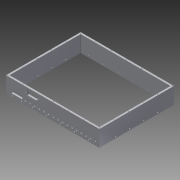
# Autodesk Inventor part: R58010-175-with SNAP V2 features
Saved by Autodesk Inventor 2016 (Build 200138000, 138)
## iProperties
Created: 2014-01-15
Part Number: R58010-175-with SNAP V2 features
Material: Aluminum 6061
Document SubType Name: Modeling
Designer: rtreacy
Density: 1 g/cm^3
Appearance: Aluminum - Flat
Author: rtreacy
Autodesk Inventor part; units mm, degrees
note: some values were not read from the file. Chosen so that the rebuilt part matches the saved one: direction of "Hole23".
ref_plane "YZ Plane" through (0, 0, 0) normal (1, 0, 0) x (0, 1, 0)
ref_plane "XZ Plane" through (0, 0, 0) normal (0, 1, 0) x (-1, 0, 0)
ref_plane "XY Plane" through (0, 0, 0) normal (0, 0, 1) x (1, 0, 0)
sketch "Ext-Sketch" plane through (0, 0, 0) normal (0, 1, 0) x (-1, 0, 0)
  line L0 (-60.3663, -75.973) -> (184.1341, -75.973)
  line L1 (184.1341, -75.973) -> (184.1341, -269.6734)
  line L2 (184.1341, -269.6734) -> (-60.3663, -269.6734)
  line L3 (-60.3663, -269.6734) -> (-60.3663, -75.973)
  line L4 (188.8839, -274.4232) -> (-65.1161, -274.4232)
  line L5 (-65.1161, -274.4232) -> (-65.1161, -71.2232)
  line L6 (-65.1161, -71.2232) -> (188.8839, -71.2232)
  line L7 (188.8839, -71.2232) -> (188.8839, -274.4232)
  point P0 (0, 0)
  dimension "d6" = 244.5004
  dimension "d8" = 193.7004
  dimension "d9" = 203.2
  dimension "d10" = 254
  dimension "d11" = 4.7498
  dimension "d12" = 4.7498
  constraints: 16 end point, 4 parallel, 2 horizontal, 2 perpendicular
  measures "d6" distance of L0.start L0.end
  measures "d8" distance of L0.end L1.end
  measures "d9" distance of L6.end L4.start
  measures "d10" distance of L4.start L4.end
  measures "d11" horizontal distance of L0.start L5.end
  measures "d12" horizontal distance of L6.end L0.end
extrude "Extrusion1" add sketch "Ext-Sketch" along normal blind 44.45
sketch "left-2" plane through (-188.8839, 0, -274.4232) normal (-1, 0, 0) x (0, 0, 1)
  circle A0 centre (19.3548, 11.938) radius 2.1971 projected
  line L0 (203.2, 0) -> (0, 0) projected
  line L1 (203.2, 0) -> (203.2, 44.45) projected
  line L2 (0, 44.45) -> (203.2, 44.45) projected
  line L3 (0, 0) -> (0, 44.45) projected
  point P0 (274.4232, 0)
sketch "left-1" plane through (-188.8839, 0, -274.4232) normal (-1, 0, 0) x (0, 0, 1)
  line L0 (4.7498, 0) -> (4.7498, 44.45) projected
  point P0 (274.4232, 0)
  point P1 (203.2, 0)
  point P2 (203.2, 44.45)
  point P3 (158.75, 4.699)
  dimension "d260" = 44.45
  dimension "d261" = 4.699
  measures "d260" horizontal distance of point (203.2, 44.45) point (158.75, 4.699)
  measures "d261" vertical distance of point (203.2, 0) point (158.75, 4.699)
sketch "bottom-1" plane through (0, 0, 0) normal (0, -1, 0) x (1, 0, 0)
  point P0 (-188.8839, -71.2232)
  point P1 (0, 0)
  point P2 (-186.509, -73.5981)
  point P3 (65.1161, -274.4232)
  point P4 (62.7412, -272.0483)
  dimension "d125" = 2.3749
  dimension "d126" = 2.3749
  dimension "d140" = 2.3749
  dimension "d141" = 2.3749
  measures "d125" horizontal distance of point (-188.884, -71.223) point (-186.509, -73.598)
  measures "d126" horizontal distance of point (-188.884, -71.223) point (-186.509, -73.598)
  measures "d140" horizontal distance of point (65.116, -274.423) point (62.741, -272.048)
  measures "d141" horizontal distance of point (65.116, -274.423) point (62.741, -272.048)
hole "Hole8" at (-186.509, 0, -73.5981) direction (0, 1, 0) diameter 1.7018 depth 5.08 tip angle 118
hole "Hole9" at (62.7412, 0, -272.0483) direction (0, 1, 0) diameter 1.7018 depth 5.08 tip angle 118
sketch "front-1" plane through (-188.8839, 0, -71.2232) normal (0, 0, 1) x (1, 0, 0)
  circle A0 centre (52.07, 10.414) radius 2.159
  line L0 (254, 0) -> (254, 44.45) projected
  line L1 (14.2748, 19.746) -> (14.2748, 9.3472)
  line L2 (14.2748, 9.3472) -> (43.975, 9.3472)
  line L3 (43.975, 9.3472) -> (43.975, 19.746)
  line L4 (43.975, 19.746) -> (14.2748, 19.746)
  line L5 (0, 44.45) -> (254, 44.45) projected
  circle A1 centre (64.77, 10.414) radius 2.159
  circle A2 centre (77.47, 10.414) radius 2.159
  circle A3 centre (90.17, 10.414) radius 2.159
  circle A4 centre (102.87, 10.414) radius 2.159
  circle A5 centre (115.57, 10.414) radius 2.159
  circle A6 centre (128.27, 10.414) radius 2.159
  circle A7 centre (140.97, 10.414) radius 2.159
  circle A8 centre (153.67, 10.414) radius 2.159
  circle A9 centre (166.37, 10.414) radius 2.159
  circle A10 centre (179.07, 10.414) radius 2.159
  circle A11 centre (191.77, 10.414) radius 2.159
  circle A12 centre (204.47, 10.414) radius 2.159
  circle A13 centre (217.17, 10.414) radius 2.159
  circle A14 centre (229.87, 10.414) radius 2.159
  circle A15 centre (242.57, 10.414) radius 2.159
  point P0 (16.51, 4.699)
  point P1 (52.07, 16.51)
  point P2 (0, 0)
  point P3 (52.07, 4.318)
  point P4 (64.77, 16.51)
  point P5 (64.77, 4.318)
  point P6 (77.47, 16.51)
  point P7 (77.47, 4.318)
  point P8 (90.17, 16.51)
  point P9 (90.17, 4.318)
  point P10 (102.87, 16.51)
  point P11 (102.87, 4.318)
  point P12 (115.57, 16.51)
  point P13 (115.57, 4.318)
  point P14 (128.27, 16.51)
  point P15 (128.27, 4.318)
  point P16 (140.97, 16.51)
  point P17 (140.97, 4.318)
  point P18 (153.67, 16.51)
  point P19 (153.67, 4.318)
  point P20 (166.37, 16.51)
  point P21 (166.37, 4.318)
  point P22 (179.07, 16.51)
  point P23 (179.07, 4.318)
  point P24 (191.77, 16.51)
  point P25 (191.77, 4.318)
  point P26 (204.47, 16.51)
  point P27 (204.47, 4.318)
  point P28 (217.17, 16.51)
  point P29 (217.17, 4.318)
  point P30 (229.87, 16.51)
  point P31 (229.87, 4.318)
  point P32 (242.57, 16.51)
  point P33 (242.57, 4.318)
  point P34 (71.12, 4.699)
  dimension "d197" = 6.096
  dimension "d203" = 12.192
  dimension "d222" = 29.7002
  dimension "d223" = 10.3988
  dimension "d224" = 52.07
  dimension "d225" = 10.414
  dimension "d227" = 9.3472
  dimension "d259" = 4.699
  dimension "d273" = 12.7
  dimension "d299" = 14.2748
  dimension "d300" = 52.07
  dimension "d301" = 52.07
  dimension "d302" = 16.51
  dimension "d306" = 6.35
  dimension "d307" = 4.699
  dimension "d434" = 4.318
  constraints: 16 centre point, 8 end point, 3 parallel, 1 horizontal, 1 perpendicular, 60 other
  measures "d197" distance of point (52.07, 16.51) A0.centre
  measures "d203" distance of point (52.07, 16.51) point (52.07, 4.318)
  measures "d222" distance of L3.end L1.start
  measures "d223" distance of L2.end L3.end
  measures "d224" horizontal distance of L5.start A0.centre
  measures "d225" vertical distance of point (0, 0) A0.centre
  measures "d227" vertical distance of L0.start L2.end
  measures "d259" vertical distance of L0.start point (16.51, 4.699)
  measures "d273" distance of point (52.07, 16.51) point (64.77, 16.51)
  measures "d299" horizontal distance of L1.start L5.start
  measures "d300" horizontal distance of point (52.07, 16.51) L5.start
  measures "d301" horizontal distance of point (52.07, 4.318) L5.start
  measures "d302" horizontal distance of point (16.51, 4.699) point (0, 0)
  measures "d306" horizontal distance of point (71.12, 4.699) A1.centre
  measures "d307" vertical distance of point (0, 0) point (71.12, 4.699)
  measures "d434" diameter of A2
hole "Hole10" at (-172.3739, 4.699, -71.2232) direction (0, 0, -1) diameter 2.4384 depth 25.4 tip angle 118 countersink diameter 4.064 countersink angle 82
sketch "right-1" plane through (65.1161, 0, -71.2232) normal (1, 0, 0) x (0, 0, -1)
  point P0 (-71.2232, 0)
  point P1 (158.75, 4.699)
  point P2 (0, 0)
  point P3 (203.2, 44.45)
  dimension "d254" = 44.45
  dimension "d255" = 4.699
  measures "d254" horizontal distance of point (203.2, 44.45) point (158.75, 4.699)
  measures "d255" vertical distance of point (0, 0) point (158.75, 4.699)
hole "Hole11" at (65.1161, 4.699, -229.9732) direction (-1, 0, 0) diameter 2.4384 depth 25.4 tip angle 118 countersink diameter 4.064 countersink angle 82
sketch "back-1" plane through (65.1161, 0, -274.4232) normal (0, 0, -1) x (-1, 0, 0)
  point P0 (65.1161, 0)
  point P1 (228.6, 4.699)
  point P2 (254, 0)
  point P3 (254, 44.45)
  dimension "d256" = 25.4
  dimension "d257" = 4.699
  measures "d256" horizontal distance of point (254, 44.45) point (228.6, 4.699)
  measures "d257" vertical distance of point (254, 0) point (228.6, 4.699)
hole "Hole12" at (-163.4839, 4.699, -274.4232) direction (0, 0, 1) diameter 2.4384 depth 25.4 tip angle 118 countersink diameter 4.064 countersink angle 82
pattern_linear "Rectangular Pattern9" count 6 spacing 39.6748 along (0, 0, -1) of "Hole8"
pattern_linear "Rectangular Pattern10" count 7 spacing 41.529 along (1, 0, 0) of "Hole8"
pattern_linear "Rectangular Pattern11" count 6 spacing 39.6748 along (0, 0, 1) of "Hole9"
pattern_linear "Rectangular Pattern12" count 7 spacing 41.529 along (-1, 0, 0) of "Hole9"
sketch "top" plane through (0, 44.45, 0) normal (0, 1, 0) x (1, 0, 0)
  point P0 (-188.8839, 274.4232)
  point P1 (0, 0)
  point P2 (-186.4709, 272.0102)
  point P3 (65.1161, 184.1791)
  dimension "d176" = 2.413
  dimension "d177" = 2.413
  measures "d176" horizontal distance of point (-188.884, 274.423) point (-186.471, 272.01)
  measures "d177" horizontal distance of point (-188.884, 274.423) point (-186.471, 272.01)
hole "Hole13" at (-186.4709, 44.45, -272.0102) direction (0, -1, 0) diameter 1.7018 depth 5.08 tip angle 118
hole "Hole16" at (-136.8139, 16.51, -71.2232) at (-136.8139, 4.318, -71.2232) direction (0, 0, -1) diameter 1.7018 depth 25.4 tip angle 118
hole "Hole17" at (-136.8139, 10.414, -71.2232) direction (0, 0, -1) diameter 4.318 depth 25.4 tip angle 118
extrude "Extrusion2" cut sketch "front-1" against normal blind 25.4 contours L4 L3 L2 L1
hole "Hole18" at (-188.8839, 4.699, -115.6732) direction (1, 0, 0) diameter 2.4384 depth 25.4 tip angle 118 countersink diameter 4.064 countersink angle 82
hole "Hole19" at (-124.1139, 10.414, -71.2232) at (-111.4139, 10.414, -71.2232) at (-98.7139, 10.414, -71.2232) at (-86.0139, 10.414, -71.2232) at (-73.3139, 10.414, -71.2232) at (-60.6139, 10.414, -71.2232) at (-47.9139, 10.414, -71.2232) at (-35.2139, 10.414, -71.2232) at (-22.5139, 10.414, -71.2232) direction (0, 0, -1) diameter 4.318 depth 25.4 tip angle 118
hole "Hole20" at (-9.8139, 10.414, -71.2232) at (2.8861, 10.414, -71.2232) at (15.5861, 10.414, -71.2232) at (28.2861, 10.414, -71.2232) at (40.9861, 10.414, -71.2232) at (53.6861, 10.414, -71.2232) direction (0, 0, -1) diameter 4.318 depth 25.4 tip angle 118
hole "Hole21" at (-124.1139, 16.51, -71.2232) at (-124.1139, 4.318, -71.2232) at (-111.4139, 16.51, -71.2232) at (-111.4139, 4.318, -71.2232) at (-98.7139, 16.51, -71.2232) at (-98.7139, 4.318, -71.2232) at (-86.0139, 16.51, -71.2232) at (-86.0139, 4.318, -71.2232) at (-73.3139, 16.51, -71.2232) at (-73.3139, 4.318, -71.2232) at (-60.6139, 16.51, -71.2232) at (-60.6139, 4.318, -71.2232) at (-47.9139, 16.51, -71.2232) at (-47.9139, 4.318, -71.2232) at (-35.2139, 16.51, -71.2232) at (-35.2139, 4.318, -71.2232) at (-22.5139, 16.51, -71.2232) at (-22.5139, 4.318, -71.2232) at (-9.8139, 16.51, -71.2232) at (-9.8139, 4.318, -71.2232) at (2.8861, 16.51, -71.2232) at (2.8861, 4.318, -71.2232) at (15.5861, 16.51, -71.2232) at (15.5861, 4.318, -71.2232) at (28.2861, 16.51, -71.2232) at (28.2861, 4.318, -71.2232) at (40.9861, 16.51, -71.2232) at (40.9861, 4.318, -71.2232) at (53.6861, 16.51, -71.2232) at (53.6861, 4.318, -71.2232) direction (0, 0, -1) diameter 1.7018 depth 5.08 tip angle 118
pattern_linear "Rectangular Pattern13" count 2 spacing 25.4 along (1, 0, 0) of "Hole10"
hole "Hole22" at (-117.7639, 4.699, -71.2232) direction (0, 0, -1) diameter 2.4384 depth 25.4 tip angle 118 countersink diameter 4.064 countersink angle 82
pattern_linear "Rectangular Pattern14" count 5 spacing 38.1 along (1, 0, 0) of "Hole22"
pattern_linear "Rectangular Pattern15" count 6 spacing 40.64 along (1, 0, 0) of "Hole12"
pattern_linear "Rectangular Pattern16" count 4 spacing 38.1 along (0, 0, 1) of "Hole11"
pattern_linear "Rectangular Pattern17" count 4 spacing 38.1 along (0, 0, -1) of "Hole18"
pattern_linear "Rectangular Pattern19" count 6 spacing 39.6748 along (0, 0, 1) count 7 spacing 41.529 along (1, 0, 0) of "Hole13"
fillet "Fillet1" radius 1.524 1 edges at (-184.1341, 22.225, -269.6734)
fillet "Fillet2" radius 1.524 1 edges at (-184.1341, 22.225, -75.973)
fillet "Fillet3" radius 1.524 1 edges at (60.3663, 22.225, -75.973)
fillet "Fillet4" radius 1.524 1 edges at (60.3663, 22.225, -269.6734)
fillet "Fillet5" radius 0.7874 1 edges at (-174.6091, 9.3472, -73.5981)
fillet "Fillet6" radius 0.7874 1 edges at (-144.9089, 9.3472, -73.5981)
fillet "Fillet7" radius 0.7874 1 edges at (-144.9089, 19.746, -73.5981)
fillet "Fillet8" radius 0.7874 1 edges at (-174.6091, 19.746, -73.5981)
sketch "front-2" plane through (-188.8839, 0, -71.2232) normal (0, 0, 1) x (1, 0, 0)
  line L0 (15.0622, 19.746) -> (43.1876, 19.746) projected
  line L1 (0, 44.45) -> (254, 44.45) projected
  line L2 (29.1249, 19.746) -> (29.1249, 44.45) construction
  circle A0 centre (71.12, 4.699) radius 2.032 projected
  line L3 (71.12, 4.699) -> (71.12, 44.45) construction
  line L4 (254, 0) -> (0, 0) projected
  line L5 (0, 0) -> (0, 44.45) projected
  line L6 (87.7824, 32.131) -> (54.4576, 32.131) construction
  arc A1 (57.9628, 37.973) -> (55.9007, 35.4264) centre (57.9628, 35.8648) ccw
  arc A2 (57.4882, 27.9588) -> (59.5503, 26.289) centre (59.5503, 28.3972) ccw
  arc A3 (86.3393, 35.4264) -> (84.2772, 37.973) centre (84.2772, 35.8648) ccw
  arc A4 (82.6897, 26.289) -> (84.7518, 27.9588) centre (82.6897, 28.3972) ccw
  line L7 (55.9007, 35.4264) -> (57.4882, 27.9588)
  line L8 (57.9628, 37.973) -> (84.2772, 37.973)
  line L9 (86.3393, 35.4264) -> (84.7518, 27.9588)
  line L10 (82.6897, 26.289) -> (59.5503, 26.289)
  point P0 (188.8839, 0)
  point P1 (71.12, 32.131)
  point P2 (71.12, 32.131)
  dimension "d372" = 33.3248
  dimension "d412" = 32.131
  dimension "d413" = 54.4576
  dimension "d414" = 4.2164
  dimension "d415" = 4.2164
  dimension "d416" = 4.2164
  dimension "d417" = 4.2164
  dimension "d418" = 11.5697
  dimension "d419" = 11.5697
  dimension "d420" = 3.7338
  dimension "d421" = 3.7338
  dimension "d422" = 13.1572
  dimension "d423" = 13.1572
  dimension "d424" = 3.7338
  dimension "d425" = 3.7338
  constraints: 14 end point, 8 point on circle, 8 tangent, 4 centre point, 3 perpendicular, 2 midpoint, 2 point on line, 1 coincident
  measures "d372" distance of L6.start L6.end
  measures "d412" distance between parallel lines of L4 L6
  measures "d413" horizontal distance of L4.end L6.end
  measures "d414" diameter of A1
  measures "d415" diameter of A2
  measures "d416" diameter of A4
  measures "d417" diameter of A3
  measures "d418" horizontal distance of point (71.12, 32.131) A2.centre
  measures "d419" horizontal distance of point (71.12, 32.131) A4.centre
  measures "d420" vertical distance of L6.end A2.centre
  measures "d421" vertical distance of L6.end A1.centre
  measures "d422" horizontal distance of point (71.12, 32.131) A1.centre
  measures "d423" horizontal distance of point (71.12, 32.131) A3.centre
  measures "d424" vertical distance of L6.start A3.centre
  measures "d425" vertical distance of L6.start A4.centre
hole "Hole23" at (-134.4263, 32.131, -71.2232) at (-101.1015, 32.131, -71.2232) direction (0, 0, -1) diameter 3.048 end up to surface
extrude "Extrusion5" cut sketch "front-2" against normal up to surface (4.7498 mm away) contours L8 A3 L9 A4 L10 A2 L7 A1
body "Solid1"
